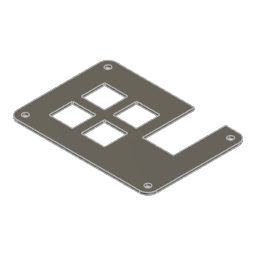
TopPartVibePad (Autodesk Fusion 360 design; units mm, degrees)
Autodesk Fusion 360 part; units mm, degrees
sketch "Esboço1" plane through (0, 0, 0) normal (0, 0, 1) x (1, 0, 0)
  line L0 (3.025, -2.525) -> (16.025, -2.525)
  line L1 (3.025, -16.525) -> (16.025, -16.525)
  line L2 (2.525, -3.025) -> (2.525, -16.025)
  line L3 (16.525, -3.025) -> (16.525, -16.025)
  arc A0 (3.025, -2.525) -> (2.525, -3.025) centre (3.025, -3.025) ccw
  arc A1 (16.525, -3.025) -> (16.025, -2.525) centre (16.025, -3.025) ccw
  arc A2 (2.525, -16.025) -> (3.025, -16.525) centre (3.025, -16.025) ccw
  arc A3 (16.025, -16.525) -> (16.525, -16.025) centre (16.025, -16.025) ccw
  line L4 (22.075, -2.525) -> (35.075, -2.525)
  line L5 (22.075, -16.525) -> (35.075, -16.525)
  line L6 (21.575, -3.025) -> (21.575, -16.025)
  line L7 (35.575, -3.025) -> (35.575, -16.025)
  arc A4 (22.075, -2.525) -> (21.575, -3.025) centre (22.075, -3.025) ccw
  arc A5 (35.575, -3.025) -> (35.075, -2.525) centre (35.075, -3.025) ccw
  arc A6 (21.575, -16.025) -> (22.075, -16.525) centre (22.075, -16.025) ccw
  arc A7 (35.075, -16.525) -> (35.575, -16.025) centre (35.075, -16.025) ccw
  line L8 (3.025, -21.575) -> (16.025, -21.575)
  line L9 (3.025, -35.575) -> (16.025, -35.575)
  line L10 (2.525, -22.075) -> (2.525, -35.075)
  line L11 (16.525, -22.075) -> (16.525, -35.075)
  arc A8 (3.025, -21.575) -> (2.525, -22.075) centre (3.025, -22.075) ccw
  arc A9 (16.525, -22.075) -> (16.025, -21.575) centre (16.025, -22.075) ccw
  arc A10 (2.525, -35.075) -> (3.025, -35.575) centre (3.025, -35.075) ccw
  arc A11 (16.025, -35.575) -> (16.525, -35.075) centre (16.025, -35.075) ccw
  line L12 (22.075, -21.575) -> (35.075, -21.575)
  line L13 (22.075, -35.575) -> (35.075, -35.575)
  line L14 (21.575, -22.075) -> (21.575, -35.075)
  line L15 (35.575, -22.075) -> (35.575, -35.075)
  arc A12 (22.075, -21.575) -> (21.575, -22.075) centre (22.075, -22.075) ccw
  arc A13 (35.575, -22.075) -> (35.075, -21.575) centre (35.075, -22.075) ccw
  arc A14 (21.575, -35.075) -> (22.075, -35.575) centre (22.075, -35.075) ccw
  arc A15 (35.075, -35.575) -> (35.575, -35.075) centre (35.075, -35.075) ccw
  line L16 (-9.475, -47.575) -> (73.425, -47.575)
  line L17 (73.425, -47.575) -> (73.425, 11.525)
  line L18 (73.425, 11.525) -> (-9.475, 11.525)
  line L19 (-9.475, 11.525) -> (-9.475, -47.575)
  line L20 (41.975, 11.525) -> (60.475, 11.525)
  line L21 (60.475, 11.525) -> (60.475, -19.475)
  line L22 (60.475, -19.475) -> (41.975, -19.475)
  line L23 (41.975, -19.475) -> (41.975, 11.525)
  circle A16 centre (68.425, -42.575) radius 1.7
  circle A17 centre (68.425, 6.525) radius 1.7
  circle A18 centre (-4.475, 6.525) radius 1.7
  circle A19 centre (-4.475, -42.575) radius 1.7
  dimension "d1" = 82.9
  dimension "d2" = 59.1
  dimension "d5" = 12
  dimension "d6" = 12
  dimension "d7" = 18.5
  dimension "d8" = 31
  dimension "d9" = 12.95
  dimension "d10" = 3.4
  dimension "d11" = 3.4
  dimension "d12" = 3.4
  dimension "d13" = 3.4
  dimension "d14" = 5
  dimension "d15" = 5
  dimension "d16" = 5
  dimension "d17" = 5
  dimension "d18" = 5
  dimension "d19" = 5
  dimension "d20" = 5
  dimension "d21" = 5
  constraint horizontal L16
  constraint vertical L17
  constraint horizontal L18
  constraint vertical L19
  constraint horizontal L20
  constraint vertical L21
  constraint horizontal L22
  constraint vertical L23
  constraint coincident L18 L20.start
  measures "d1" distance of L16.start L16.end
  measures "d2" distance of L16.start L18.end
  measures "d5" distance of L10 L19
  measures "d6" distance of L9 L16
  measures "d7" distance of L20.start L20.end
  measures "d8" distance of L20.start L22.end
  measures "d9" distance of L17 L21
  measures "d10" diameter of A16
  measures "d11" diameter of A17
  measures "d12" diameter of A18
  measures "d13" diameter of A19
  measures "d14" distance of L16 A19.centre
  measures "d15" distance of L19 A19.centre
  measures "d16" distance of L17 A16.centre
  measures "d17" distance of L16 A16.centre
  measures "d18" distance of L17 A17.centre
  measures "d19" distance of L18 A17.centre
  measures "d20" distance of L18 A18.centre
  measures "d21" distance of L19 A18.centre
extrude "Extrusão1" add sketch "Esboço1" along normal blind 1.5 contours L16 L17 L18 L19 L21 L22 L23
fillet "Arredondamento1" radius 5 4 edges at (73.425, -47.575, 0.75) (73.425, 11.525, 0.75) (-9.475, 11.525, 0.75) (-9.475, -47.575, 0.75)
sketch "Esboço2" plane through (0, 0, 0) normal (0, 0, -1) x (1, 0, 0)
  arc A0 (2.525, 3.025) -> (3.025, 2.525) centre (3.025, 3.025) ccw
  line L0 (2.525, 3.025) -> (2.525, 16.025)
  arc A1 (3.025, 16.525) -> (2.525, 16.025) centre (3.025, 16.025) ccw
  line L1 (3.025, 16.525) -> (16.025, 16.525)
  arc A2 (16.525, 16.025) -> (16.025, 16.525) centre (16.025, 16.025) ccw
  line L2 (16.525, 16.025) -> (16.525, 3.025)
  arc A3 (16.025, 2.525) -> (16.525, 3.025) centre (16.025, 3.025) ccw
  line L3 (16.025, 2.525) -> (3.025, 2.525)
  arc A4 (2.525, 22.075) -> (3.025, 21.575) centre (3.025, 22.075) ccw
  line L4 (2.525, 22.075) -> (2.525, 35.075)
  arc A5 (3.025, 35.575) -> (2.525, 35.075) centre (3.025, 35.075) ccw
  line L5 (3.025, 35.575) -> (16.025, 35.575)
  arc A6 (16.525, 35.075) -> (16.025, 35.575) centre (16.025, 35.075) ccw
  line L6 (16.525, 35.075) -> (16.525, 22.075)
  arc A7 (16.025, 21.575) -> (16.525, 22.075) centre (16.025, 22.075) ccw
  line L7 (16.025, 21.575) -> (3.025, 21.575)
  circle A8 centre (68.425, -6.525) radius 1.7
  circle A9 centre (68.425, 42.575) radius 1.7
  arc A10 (21.575, 22.075) -> (22.075, 21.575) centre (22.075, 22.075) ccw
  line L8 (21.575, 22.075) -> (21.575, 35.075)
  arc A11 (22.075, 35.575) -> (21.575, 35.075) centre (22.075, 35.075) ccw
  line L9 (22.075, 35.575) -> (35.075, 35.575)
  arc A12 (35.575, 35.075) -> (35.075, 35.575) centre (35.075, 35.075) ccw
  line L10 (35.575, 35.075) -> (35.575, 22.075)
  arc A13 (35.075, 21.575) -> (35.575, 22.075) centre (35.075, 22.075) ccw
  line L11 (35.075, 21.575) -> (22.075, 21.575)
  circle A14 centre (-4.475, 42.575) radius 1.7
  arc A15 (21.575, 3.025) -> (22.075, 2.525) centre (22.075, 3.025) ccw
  line L12 (21.575, 3.025) -> (21.575, 16.025)
  arc A16 (22.075, 16.525) -> (21.575, 16.025) centre (22.075, 16.025) ccw
  line L13 (22.075, 16.525) -> (35.075, 16.525)
  arc A17 (35.575, 16.025) -> (35.075, 16.525) centre (35.075, 16.025) ccw
  line L14 (35.575, 16.025) -> (35.575, 3.025)
  arc A18 (35.075, 2.525) -> (35.575, 3.025) centre (35.075, 3.025) ccw
  line L15 (35.075, 2.525) -> (22.075, 2.525)
  circle A19 centre (-4.475, -6.525) radius 1.7
  arc A20 (-4.475, 47.575) -> (-9.475, 42.575) centre (-4.475, 42.575) ccw
  line L16 (-9.475, 42.575) -> (-9.475, -6.525)
  arc A21 (-9.475, -6.525) -> (-4.475, -11.525) centre (-4.475, -6.525) ccw
  line L17 (-4.475, -11.525) -> (41.975, -11.525)
  line L18 (41.975, -11.525) -> (41.975, 19.475)
  line L19 (41.975, 19.475) -> (60.475, 19.475)
  line L20 (60.475, 19.475) -> (60.475, -11.525)
  line L21 (60.475, -11.525) -> (68.425, -11.525)
  arc A22 (68.425, -11.525) -> (73.425, -6.525) centre (68.425, -6.525) ccw
  line L22 (73.425, -6.525) -> (73.425, 42.575)
  arc A23 (73.425, 42.575) -> (68.425, 47.575) centre (68.425, 42.575) ccw
  line L23 (68.425, 47.575) -> (-4.475, 47.575)
  line L24 (40.508, 28.482) -> (61.6076, 28.7076) construction
  line L25 (61.6076, 28.7076) -> (61.492, 39.518) construction
  line L26 (61.492, 39.518) -> (40.3924, 39.2924) construction
  line L27 (40.3924, 39.2924) -> (40.508, 28.482) construction
  dimension "d26" = 2
  text T0 "VibePad Gaming\nMade by Nix\n\nWith the help of:\nhackclub.com" font "Arial" height 2 align left top in box 21.1007 x 10.8111 at (40.508, 28.482) x (0.999943, 0.010692) y (-0.010692, 0.999943) spacing 1 kerned
extrude "Extrusão2" add sketch "Esboço2" along normal blind 0.2 text T0
equation "d27 = 'VibePad Gaming Made by Nix With the help of: hackclub.com'"
